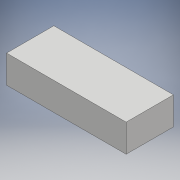
# Autodesk Inventor part: waterblock connector
Saved by Autodesk Inventor 2018 (Build 220112000, 112)
## iProperties
Created: 2018-06-21
Part Number: waterblock connector
Material: Generic
Document SubType Name: Modeling
Designer: John Viljoen
Density: 1 g/cm^3
Appearance: Default
Author: John Viljoen
Autodesk Inventor part; units mm, degrees
ref_plane "YZ Plane" through (0, 0, 0) normal (1, 0, 0) x (0, 1, 0)
ref_plane "XZ Plane" through (0, 0, 0) normal (0, 1, 0) x (-1, 0, 0)
ref_plane "XY Plane" through (0, 0, 0) normal (0, 0, 1) x (1, 0, 0)
sketch "Sketch1" plane through (0, 0, 0) normal (0, 0, 1) x (1, 0, 0)
  line L0 (0, 0) -> (64.5, 0)
  line L1 (64.5, 0) -> (64.5, 25.5)
  line L2 (64.5, 25.5) -> (0, 25.5)
  line L3 (0, 25.5) -> (0, 0)
  dimension "d0" = 64.5
  dimension "d1" = 25.5
  constraints: 8 end point, 2 parallel, 1 horizontal, 1 perpendicular
  measures "d0" distance of L2.end L1.end
  measures "d1" distance of L1.end L0.end
extrude "Extrusion1" add sketch "Sketch1" along normal blind 15
body "Solid1"
